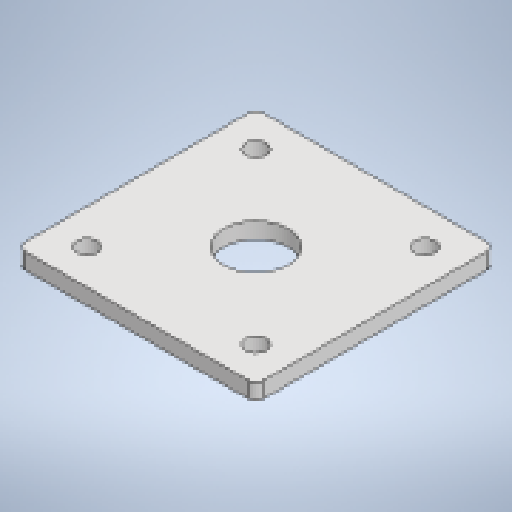
# Autodesk Inventor part: NVPH-343 cup head flange
Saved by Autodesk Inventor 2025.1 (Build 291241020, 241B)
## iProperties
Created: 2024-12-03
Part Number: NVPH-343 cup head flange
Material: Generic
Document SubType Name: Sheet Metal
Designer: user
Density: 1 g/cm^3
Flat Pattern Width: 17 cm
Flat Pattern Length: 17 cm
Flat Pattern Area: 289 cm^2
Sheet Metal Rule: Default_mm
Sheet Metal Width: 170.000 mm
Sheet Metal Length: 170.000 mm
Sheet Metal Area: 28900.000 mm^2
Appearance: Default
Mass: 294.807 g
Surface Area: 687.632 cm^2
Volume: 294.807 cm^3
Author: user
Autodesk Inventor part; units mm, degrees
ref_plane "YZ Plane" through (0, 0, 0) normal (1, 0, 0) x (0, 1, 0)
ref_plane "XZ Plane" through (0, 0, 0) normal (0, 1, 0) x (-1, 0, 0)
ref_plane "XY Plane" through (0, 0, 0) normal (0, 0, 1) x (1, 0, 0)
sketch "Sketch1" plane through (0, 0, 0) normal (0, 0, 1) x (1, 0, 0)
  circle A0 centre (0, 0) radius 20
  line L0 (-85, -85) -> (85, -85)
  line L1 (85, -85) -> (85, 85)
  line L2 (85, 85) -> (-85, 85)
  line L3 (-85, 85) -> (-85, -85)
  line L4 (-85, -85) -> (85, 85) construction
  line L5 (85, -85) -> (-85, 85) construction
  dimension "d0" = 40
  dimension "d13" = 170
  constraints: 12 end point, 2 midpoint, 2 parallel, 2 perpendicular, 1 centre point, 1 coincident, 1 horizontal
  measures "d0" diameter of A0
  measures "d13" distance of L2.end L0.start
extrude "Extrusion1" add sketch "Sketch1" against normal blind 10
sketch "Sketch4" plane through (0, 0, 0) normal (0, 0, 1) x (1, 0, 0)
  line L0 (85, 85) -> (-85, 85) projected
  line L1 (-85, -85) -> (85, -85) projected
  line L2 (0, 0) -> (85, 85) construction
  circle A0 centre (67.1751, 67.1751) radius 6.5
  circle A1 centre (0, 0) radius 95 construction
  dimension "d22" = 190
  dimension "d23" = 13
  constraints: 2 end point, 1 centre point, 1 coincident, 1 point on line, 3 other
  measures "d23" diameter of A0
extrude "Extrusion2" cut sketch "Sketch4" against normal through all
pattern_circular "Circular Pattern2" count 4 over 360 about axis through (0, 0, 0) along (0, 0, -1) of "Extrusion2"
fillet "Fillet1" radius 5 4 edges at (85, -85, -5) (-85, -85, -5) (-85, 85, -5) (85, 85, -5)
equation "\"BendReliefDepth\" = 0.5 * Thickness"
equation "\"Thickness\" = 10"
body "Solid1"
